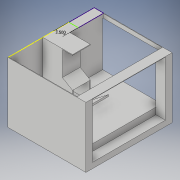
# Autodesk Inventor part: bot test 1
Saved by Autodesk Inventor 2018 (Build 220112000, 112)
## iProperties
Created: 2017-10-21
Part Number: bot test 1
Material: Generic
Document SubType Name: Modeling
Designer: 17firish
Density: 1 g/cm^3
Appearance: Default
Author: 17firish
Autodesk Inventor part; units mm, degrees
ref_plane "YZ Plane" through (0, 0, 0) normal (1, 0, 0) x (0, 1, 0)
ref_plane "XZ Plane" through (0, 0, 0) normal (0, 1, 0) x (-1, 0, 0)
ref_plane "XY Plane" through (0, 0, 0) normal (0, 0, 1) x (1, 0, 0)
sketch "Sketch1" plane through (0, 0, 0) normal (0, 1, 0) x (-1, 0, 0)
  line L0 (0, 0) -> (-736.6, 0)
  line L1 (-736.6, 0) -> (-736.6, -812.8)
  line L2 (-736.6, -812.8) -> (0, -812.8)
  line L3 (0, -812.8) -> (0, 0)
  dimension "d0" = 736.6
  dimension "d1" = 812.8
  constraints: 8 end point, 2 parallel, 1 horizontal, 1 perpendicular
  measures "d0" distance of L2.end L1.end
  measures "d1" distance of L1.end L0.end
extrude "Extrusion1" add sketch "Sketch1" along normal blind 571.5
sketch "Sketch2" plane through (0, 571.5, 0) normal (0, 1, 0) x (1, 0, 0)
  line L0 (0, 812.8) -> (0, 0) projected
  line L1 (0, 812.8) -> (88.9, 812.8)
  line L2 (88.9, 812.8) -> (88.9, 574.8444)
  line L3 (88.9, 574.8444) -> (0, 574.8444)
  line L4 (0, 574.8444) -> (0, 812.8)
  dimension "d4" = 88.9
  constraints: 8 end point, 2 parallel, 1 horizontal, 1 perpendicular
  measures "d4" distance of L2.end L3.end
sketch "Sketch7" plane through (0, 571.5, 0) normal (0, 1, 0) x (1, 0, 0)
  line L0 (647.7, 808.0248) -> (90.8173, 808.0248)
  line L1 (90.8173, 808.0248) -> (90.8173, 495.3)
  line L2 (0, 327.5313) -> (279.4, 327.5313)
  line L3 (282.5115, 327.5313) -> (282.5115, 495.3)
  line L4 (279.4, 327.5313) -> (282.5115, 327.5313)
  line L5 (282.5115, 327.5313) -> (0, 327.5313)
  line L6 (647.7, 808.0248) -> (90.8173, 808.0248)
  line L7 (282.5115, 495.3) -> (90.8173, 495.3)
  line L8 (1.5741, 327.5313) -> (1.5741, 4.7643)
  line L9 (1.5741, 4.7643) -> (647.7, 5.5504)
  line L10 (647.7, 808.0248) -> (647.7, 5.5504)
  line L11 (0, 0) -> (736.6, 0) projected
  point P0 (736.6, 812.8)
  constraints: 22 end point, 1 collinear, 1 horizontal, 1 perpendicular, 1 point on line
extrude "Extrusion7" cut sketch "Sketch7" against normal blind 457.2
sketch "Sketch8" plane through (736.6, 0, 0) normal (1, 0, 0) x (0, 0, -1)
  line L0 (60.9734, 567.6333) -> (749.1017, 567.6333)
  line L1 (749.1017, 567.6333) -> (749.1017, 52.2629)
  line L2 (749.1017, 52.2629) -> (60.9734, 52.2629)
  line L3 (60.9734, 52.2629) -> (60.9734, 567.6333)
  point P0 (0, 0)
  constraints: 8 end point, 2 parallel, 1 horizontal, 1 perpendicular
extrude "Extrusion8" cut sketch "Sketch8" against normal blind 88.9
sketch "Sketch9" plane through (282.5115, 571.5, -327.5313) normal (1, 0, 0) x (0, 0, -1)
  line L0 (0, 0) -> (0, -457.2) projected
  line L1 (0, -292.1) -> (167.7687, -292.1)
  line L2 (167.7687, 0) -> (167.7687, -457.2) projected
  line L3 (421.5704, -457.2) -> (-266.5579, -457.2) projected
  line L4 (9.1846, -292.1) -> (9.1846, -457.2)
  line L5 (160.1669, -292.1) -> (160.1669, -457.2)
  point P0 (-327.5313, -571.5)
  dimension "d29" = 165.1
  constraints: 6 end point, 6 point on line, 2 perpendicular, 1 horizontal
  measures "d29" distance between parallel lines of L3 L1
extrude "Extrusion9" cut sketch "Sketch9" against normal blind 192.0875 contours L1 L5 L3 L4
sketch "Sketch10" plane through (736.6, 0, -812.8) normal (0, 0, -1) x (-1, 0, 0)
  line L0 (88.9, 571.5) -> (88.9, 114.3) projected
  line L1 (88.9, 532.7914) -> (711.9203, 532.7914)
  line L2 (711.9203, 532.7914) -> (711.9203, 34.8419)
  line L3 (711.9203, 34.8419) -> (88.9, 34.8419)
  line L4 (88.9, 34.8419) -> (88.9, 532.7914)
  point P0 (736.6, 0)
  constraints: 8 end point, 2 parallel, 1 horizontal, 1 perpendicular, 1 point on line
extrude "Extrusion10" cut sketch "Sketch10" against normal blind 9.525
sketch "Sketch11" plane through (282.5115, 571.5, -495.3) normal (0, 0, -1) x (-1, 0, 0)
  line L0 (0, 0) -> (0, -457.2) projected
  line L1 (0, -292.1) -> (191.6942, -292.1)
  line L2 (191.6942, 0) -> (191.6942, -457.2) projected
  line L3 (0, -457.2) -> (191.6942, -457.2) projected
  line L4 (95.25, -292.1) -> (95.25, -234.95)
  line L5 (0, -292.1) -> (95.25, -234.95)
  line L6 (95.25, -234.95) -> (95.25, -6.35)
  line L7 (95.25, -6.35) -> (0, -6.35)
  point P0 (282.5115, -571.5)
  dimension "d34" = 165.1
  dimension "d35" = 57.15
  dimension "d36" = 95.25
  dimension "d37" = 228.6
  constraints: 10 end point, 4 point on line, 2 vertical, 1 horizontal, 1 perpendicular
  measures "d34" distance between parallel lines of L3 L1
  measures "d35" distance of L4.start L4.end
  measures "d36" distance between parallel lines of L0 L4
  measures "d37" distance of L4.end L6.end
extrude "Extrusion11" cut sketch "Sketch11" against normal blind 192.0875 contours L7 L6 L5 L0
sketch "Sketch12" plane through (0, 114.3, 0) normal (0, 1, 0) x (1, 0, 0)
  line L0 (282.5115, 336.7158) -> (460.3115, 336.7158)
  line L1 (460.3115, 336.7158) -> (460.3115, 487.6982)
  line L2 (460.3115, 487.6982) -> (282.5115, 487.6982)
  line L3 (282.5115, 487.6982) -> (282.5115, 336.7158)
  point P0 (0, 0)
  dimension "d40" = 177.8
  constraints: 8 end point, 2 parallel, 1 horizontal, 1 perpendicular
  measures "d40" distance of L2.end L1.end
extrude "Extrusion12" add sketch "Sketch12" along normal blind 139.7
sketch "Sketch13" plane through (460.3115, 114.3, -487.6982) normal (0, 0, -1) x (-1, 0, 0)
  line L0 (0, 0) -> (0, 139.7) projected
  line L1 (177.8, 165.1) -> (177.8, 0) projected
  line L2 (0, 139.7) -> (177.8, 0)
  line L3 (0, 122.6899) -> (156.1508, 0)
  line L4 (-187.3885, 0) -> (369.4942, 0) projected
  point P0 (460.3115, -114.3)
  constraints: 4 end point, 2 point on line, 1 parallel
extrude "Extrusion13" cut sketch "Sketch13" against normal blind 188.9125 contours L0 L3 L4
sketch "Sketch14" plane through (460.3115, 254, -487.6982) normal (0, 0, -1) x (-1, 0, 0)
  line L0 (177.8, 0) -> (177.8, -139.7) projected
  line L1 (0, 0) -> (177.8, -139.7)
  line L2 (458.7374, -139.7) -> (177.8, -139.7) projected
  line L3 (177.8, -139.7) -> (177.8, 0) projected
  line L4 (177.8, -139.7) -> (177.8, 0)
  line L5 (0, 0) -> (177.8, 0) projected
  line L6 (177.8, 0) -> (0, 0)
  point P0 (460.3115, -254)
  constraints: 6 end point, 1 collinear, 1 perpendicular
extrude "Extrusion14" cut sketch "Sketch14" against normal blind 185.7375
body "Solid1"
